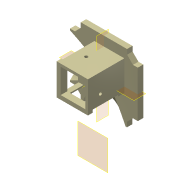
# Autodesk Inventor part: 20_Cube_Insert_Lightsheet_FEPTube_shifted_v3
Saved by Autodesk Inventor 2022 (Build 260153000, 153)
## iProperties
Created: 2019-07-01
Part Number: 20_Cube_Insert_Lightsheet_FEPTube_shifted_v3
Material: Generic
Document SubType Name: Modeling
Designer: diederichbenedict
Density: 1 g/cm^3
Appearance: Nylon 6
Author: diederichbenedict
Autodesk Inventor part; units mm, degrees
ref_plane "YZ Plane" through (0, 0, 0) normal (1, 0, 0) x (0, 1, 0)
ref_plane "XZ Plane" through (0, 0, 0) normal (0, 1, 0) x (-1, 0, 0)
ref_plane "Work Plane1" through (0, 0, 10) normal (0, 0, 1) x (1, 0, 0)
sketch "Sketch1" plane through (0, 0, 10) normal (0, 0, 1) x (1, 0, 0)
  line L0 (-4.029928, -0.353838) -> (-2.232156, 1.443934) construction
  arc A0 (-1.443934, 2.232156) -> (-2.232156, 1.443934) centre (-0.929928, 0.929928) ccw construction
  line L1 (-1.443934, 2.232156) -> (0.353838, 4.029928) construction
  line L2 (-37.829928, 42.829928) -> (-37.829928, 37.829928) construction
  line L3 (-37.829928, 37.829928) -> (-42.920801, 37.829928) construction
  line L4 (-37.829928, 42.213694) -> (-37.829928, 45.829928) construction
  line L5 (-37.829928, 45.829928) -> (-4.029928, 45.829928) construction
  line L6 (-4.029928, 45.829928) -> (-4.029928, 42.213694) construction
  line L7 (-4.029928, 4.029928) -> (0.353838, 4.029928)
  circle A1 centre (-20.929928, 20.929928) radius 17.5
  line L8 (-20.929928, 58.972273) -> (17.112417, 20.929928) construction
  line L9 (17.112417, 20.929928) -> (-20.929928, -17.112417) construction
  line L10 (-20.929928, -17.112417) -> (-58.972273, 20.929928) construction
  line L11 (-58.972273, 20.929928) -> (-20.929928, 58.972273) construction
  line L12 (-20.929928, 58.972273) -> (-20.929928, -17.112417) construction
  line L13 (17.112417, 20.929928) -> (-58.972273, 20.929928) construction
  line L14 (-20.929928, 58.972273) -> (32.870072, 58.972273) construction
  line L15 (-43.429928, 43.429928) -> (1.570072, 43.429928) construction
  line L16 (1.570072, 43.429928) -> (1.570072, -1.570072) construction
  line L17 (1.570072, -1.570072) -> (-43.429928, -1.570072) construction
  line L18 (-43.429928, -1.570072) -> (-43.429928, 43.429928) construction
  line L19 (-43.429928, 43.429928) -> (1.570072, -1.570072) construction
  line L20 (1.570072, 43.429928) -> (-43.429928, -1.570072) construction
  line L21 (-43.429928, 5.387583) -> (-43.429928, 36.472273)
  line L22 (-43.429928, 36.472273) -> (-36.472273, 43.429928)
  line L23 (-36.472273, 43.429928) -> (-5.387583, 43.429928)
  line L24 (-5.387583, 43.429928) -> (1.570072, 36.472273)
  line L25 (1.570072, 36.472273) -> (1.570072, 5.387583)
  line L26 (1.570072, 5.387583) -> (-5.387583, -1.570072)
  line L27 (-5.387583, -1.570072) -> (-36.472273, -1.570072)
  line L28 (-36.472273, -1.570072) -> (-43.429928, 5.387583)
  line L29 (-4.029928, 42.213694) -> (-37.829928, 42.213694)
  line L30 (-4.029928, -0.353838) -> (-4.029928, 4.029928)
  circle A2 centre (-20.929928, 20.929928) radius 1.5
  line L31 (-10.929928, 10.929928) -> (-30.929928, 10.929928) construction
  line L32 (-30.929928, 10.929928) -> (-30.929928, 30.929928) construction
  line L33 (-30.929928, 30.929928) -> (-10.929928, 30.929928) construction
  line L34 (-10.929928, 30.929928) -> (-10.929928, 10.929928) construction
  line L35 (-10.929928, 10.929928) -> (-30.929928, 30.929928) construction
  line L36 (-30.929928, 10.929928) -> (-10.929928, 30.929928) construction
  circle A3 centre (-30.929928, 30.929928) radius 1.4
  circle A4 centre (-30.929928, 10.929928) radius 1.4
  circle A5 centre (-10.929928, 10.929928) radius 1.4
  line L37 (-45.829928, 37.829928) -> (-42.072273, 37.829928) construction
  line L38 (-42.172273, 37.729928) -> (-45.829928, 37.729928)
  line L39 (-45.829928, 37.729928) -> (-45.829928, 4.129928)
  line L40 (-45.829928, 4.129928) -> (-42.172273, 4.129928)
  line L41 (-42.172273, 4.129928) -> (-42.172273, 37.729928)
  line L42 (-45.829928, 4.029928) -> (-42.072273, 4.029928) construction
  line L43 (-45.829928, 37.829928) -> (-42.072273, 37.829928)
  line L44 (-37.729928, 45.829928) -> (-4.129928, 45.829928)
  line L45 (-4.129928, 45.829928) -> (-4.129928, 42.172273)
  line L46 (-4.129928, 42.172273) -> (-37.729928, 42.172273)
  line L47 (-37.729928, 42.172273) -> (-37.729928, 45.829928)
  line L48 (0.470072, 37.829928) -> (0.470072, 4.029928) construction
  line L49 (0.470072, 4.029928) -> (3.970072, 4.029928) construction
  line L50 (3.970072, 37.829928) -> (3.970072, 4.029928) construction
  line L51 (0.470072, 37.829928) -> (3.970072, 37.829928) construction
  line L52 (-45.829928, -3.970072) -> (-4.029928, -3.970072) construction
  line L53 (0.312417, 37.729928) -> (3.970072, 37.729928)
  line L54 (3.970072, 37.729928) -> (3.970072, 4.129928)
  line L55 (3.970072, 4.129928) -> (0.312417, 4.129928)
  line L56 (0.312417, 4.129928) -> (0.312417, 37.729928)
  line L57 (-4.171349, -0.353838) -> (-37.729928, -0.353838)
  line L58 (-37.729928, -0.353838) -> (-37.729928, -3.970072)
  line L59 (-37.729928, -3.970072) -> (-4.171349, -3.970072)
  line L60 (-4.171349, -3.970072) -> (-4.171349, -0.353838)
  point P0 (-37.829928, 4.029928)
  dimension "d18" = 53.8
  dimension "d19" = 45
  dimension "d20" = 53.8
  dimension "d21" = 45
  dimension "d22" = 45
  dimension "d30" = 20
  dimension "d31" = 20
  dimension "d32" = 2.8
  dimension "d33" = 2.8
  dimension "d34" = 2.8
  dimension "d35" = 3
  dimension "d36" = 0.1
  dimension "d37" = 0.1
  dimension "d38" = 0.1
  dimension "d39" = 0.1
  constraints: 86 end point, 21 point on line, 14 parallel, 8 perpendicular, 7 horizontal, 7 midpoint, 4 centre point, 4 coincident, 1 equal length
  measures "d18" distance of L8.start L8.end
  measures "d19" angle of L8 L14
  measures "d20" distance of L8.end L9.end
  measures "d21" distance of L16.end L17.end
  measures "d22" distance of L15.end L16.end
  measures "d30" distance of L32.end L33.end
  measures "d31" distance of L31.end L32.end
  measures "d32" diameter of A3
  measures "d33" diameter of A4
  measures "d34" diameter of A5
  measures "d35" diameter of A2
  measures "d36" distance between parallel lines of L38 L43
  measures "d37" distance between parallel lines of L40 L42
  measures "d38" distance between parallel lines of L45 L6
  measures "d39" distance between parallel lines of L4 L47
sketch "Sketch1 outline for Extrusion1" plane through (0, 0, 10) normal (0, 0, 1) x (1, 0, 0)
  line L0 (-37.729928, -3.970072) -> (-4.171349, -3.970072)
  line L1 (-4.171349, -3.970072) -> (-4.171349, -0.353838)
  line L2 (0.312417, 4.129928) -> (-4.171349, -0.353838)
  line L3 (0.312417, 4.129928) -> (3.970072, 4.129928)
  line L4 (3.970072, 4.129928) -> (3.970072, 37.729928)
  line L5 (3.970072, 37.729928) -> (0.312417, 37.729928)
  line L6 (-4.129928, 42.172273) -> (0.312417, 37.729928)
  line L7 (-4.129928, 42.172273) -> (-4.129928, 45.829928)
  line L8 (-4.129928, 45.829928) -> (-37.729928, 45.829928)
  line L9 (-37.729928, 45.829928) -> (-37.729928, 42.172273)
  line L10 (-42.172273, 37.729928) -> (-37.729928, 42.172273)
  line L11 (-42.172273, 37.729928) -> (-45.829928, 37.729928)
  line L12 (-45.829928, 37.729928) -> (-45.829928, 4.129928)
  line L13 (-45.829928, 4.129928) -> (-42.172273, 4.129928)
  line L14 (-37.688507, -0.353838) -> (-42.172273, 4.129928)
  line L15 (-37.688507, -0.353838) -> (-37.729928, -0.353838)
  line L16 (-37.729928, -0.353838) -> (-37.729928, -3.970072)
extrude "Extrusion1" add sketch "Sketch1 outline for Extrusion1" along normal blind 3
sketch "Skizze4" plane through (0, 0, 13) normal (0, 0, 1) x (1, 0, 0)
  line L0 (-37.729928, 42.172273) -> (-42.172273, 37.729928)
  line L1 (-42.172273, 37.729928) -> (-45.829928, 37.729928)
  line L2 (-45.829928, 37.729928) -> (-45.829928, 4.129928) construction
  line L3 (-45.829928, 4.129928) -> (-42.172273, 4.129928)
  line L4 (-42.172273, 4.129928) -> (-37.688507, -0.353838)
  line L5 (-37.688507, -0.353838) -> (-37.729928, -0.353838)
  line L6 (-37.729928, -0.353838) -> (-37.729928, -3.970072)
  line L7 (-37.729928, -3.970072) -> (-4.171349, -3.970072) construction
  line L8 (-4.171349, -3.970072) -> (-4.171349, -0.353838)
  line L9 (-4.171349, -0.353838) -> (0.312417, 4.129928)
  line L10 (0.312417, 4.129928) -> (3.970072, 4.129928)
  line L11 (3.970072, 4.129928) -> (3.970072, 37.729928) construction
  line L12 (3.970072, 37.729928) -> (0.312417, 37.729928)
  line L13 (0.312417, 37.729928) -> (-4.129928, 42.172273)
  line L14 (-4.129928, 42.172273) -> (-4.129928, 45.829928)
  line L15 (-4.129928, 45.829928) -> (-37.729928, 45.829928) construction
  line L16 (-37.729928, 45.829928) -> (-37.729928, 42.172273)
  line L17 (-37.929928, 46.029928) -> (-3.929928, 46.029928) construction
  line L18 (-3.929928, 46.029928) -> (-3.929928, 42.255116)
  line L19 (-3.929928, 42.255116) -> (0.39526, 37.929928)
  line L20 (0.39526, 37.929928) -> (4.170072, 37.929928)
  line L21 (4.170072, 37.929928) -> (4.170072, 3.929928) construction
  line L22 (4.170072, 3.929928) -> (0.39526, 3.929928)
  line L23 (0.39526, 3.929928) -> (-3.971349, -0.436681)
  line L24 (-3.971349, -0.436681) -> (-3.971349, -4.170072)
  line L25 (-3.971349, -4.170072) -> (-37.929928, -4.170072) construction
  line L26 (-37.929928, -4.170072) -> (-37.929928, -0.39526)
  line L27 (-37.929928, -0.39526) -> (-42.255116, 3.929928)
  line L28 (-42.255116, 3.929928) -> (-46.029928, 3.929928)
  line L29 (-46.029928, 3.929928) -> (-46.029928, 37.929928) construction
  line L30 (-46.029928, 37.929928) -> (-42.255116, 37.929928)
  line L31 (-42.255116, 37.929928) -> (-37.929928, 42.255116)
  line L32 (-37.929928, 42.255116) -> (-37.929928, 46.029928)
  line L33 (-45.829928, 37.729928) -> (-45.829928, 37.929928)
  line L34 (-4.129928, 45.829928) -> (-37.729928, 45.829928)
  line L35 (-37.729928, 45.829928) -> (-37.929928, 45.829928)
  line L36 (-4.129928, 45.829928) -> (-3.929928, 45.829928)
  line L37 (3.970072, 37.729928) -> (3.970072, 37.929928)
  line L38 (3.970072, 4.129928) -> (3.970072, 37.729928)
  line L39 (3.970072, 4.129928) -> (3.970072, 3.929928)
  line L40 (-4.171349, -3.970072) -> (-3.971349, -3.970072)
  line L41 (-37.729928, -3.970072) -> (-37.929928, -3.970072)
  line L42 (-45.829928, 4.129928) -> (-45.829928, 3.929928)
  point P0 (0, 0)
  dimension "d40" = 0.2
  constraints: 48 end point, 12 point on line, 4 perpendicular, 15 other
  measures "d40" distance between parallel lines of L15 L17
sketch "Skizze4 outline for IM_offset" plane through (0, 0, 13) normal (0, 0, 1) x (1, 0, 0)
  line L0 (-3.929928, 45.829928) -> (-4.129928, 45.829928)
  line L1 (-3.929928, 42.255116) -> (-3.929928, 45.829928)
  line L2 (0.39526, 37.929928) -> (-3.929928, 42.255116)
  line L3 (3.970072, 37.929928) -> (0.39526, 37.929928)
  line L4 (3.970072, 37.729928) -> (3.970072, 37.929928)
  line L5 (0.312417, 37.729928) -> (3.970072, 37.729928)
  line L6 (-4.129928, 42.172273) -> (0.312417, 37.729928)
  line L7 (-4.129928, 45.829928) -> (-4.129928, 42.172273)
  line L8 (-42.172273, 37.729928) -> (-37.729928, 42.172273)
  line L9 (-45.829928, 37.729928) -> (-42.172273, 37.729928)
  line L10 (-45.829928, 37.929928) -> (-45.829928, 37.729928)
  line L11 (-42.255116, 37.929928) -> (-45.829928, 37.929928)
  line L12 (-37.929928, 42.255116) -> (-42.255116, 37.929928)
  line L13 (-37.929928, 45.829928) -> (-37.929928, 42.255116)
  line L14 (-37.729928, 45.829928) -> (-37.929928, 45.829928)
  line L15 (-37.729928, 42.172273) -> (-37.729928, 45.829928)
  line L16 (-45.829928, 4.129928) -> (-42.172273, 4.129928)
  line L17 (-42.172273, 4.129928) -> (-37.688507, -0.353838)
  line L18 (-37.688507, -0.353838) -> (-37.729928, -0.353838)
  line L19 (-37.729928, -0.353838) -> (-37.729928, -3.970072)
  line L20 (-37.729928, -3.970072) -> (-37.929928, -3.970072)
  line L21 (-37.929928, -3.970072) -> (-37.929928, -0.39526)
  line L22 (-37.929928, -0.39526) -> (-42.255116, 3.929928)
  line L23 (-42.255116, 3.929928) -> (-45.829928, 3.929928)
  line L24 (-45.829928, 3.929928) -> (-45.829928, 4.129928)
  line L25 (3.970072, 3.929928) -> (3.970072, 4.129928)
  line L26 (0.39526, 3.929928) -> (3.970072, 3.929928)
  line L27 (-3.971349, -0.436681) -> (0.39526, 3.929928)
  line L28 (-3.971349, -3.970072) -> (-3.971349, -0.436681)
  line L29 (-4.171349, -3.970072) -> (-3.971349, -3.970072)
  line L30 (-4.171349, -0.353838) -> (-4.171349, -3.970072)
  line L31 (0.312417, 4.129928) -> (-4.171349, -0.353838)
  line L32 (3.970072, 4.129928) -> (0.312417, 4.129928)
extrude "IM_offset" add sketch "Skizze4 outline for IM_offset" against normal up to surface (3 mm away)
ref_plane "Arbeitsebene5" through (-20.929928, 3.929928, 10) normal (1, 0, 0) x (0, 0, -1)
ref_plane "Arbeitsebene6" through (-37.929928, 20.929928, 10) normal (0, 1, 0) x (1, 0, 0)
sketch "Skizze25" plane through (0, 0, 13) normal (0, 0, 1) x (1, 0, 0)
  line L0 (3.970072, 3.929928) -> (3.970072, 37.929928)
  line L1 (3.970072, 37.929928) -> (0.39526, 37.929928)
  line L2 (0.39526, 37.929928) -> (-3.929928, 42.255116)
  line L3 (-3.929928, 42.255116) -> (-3.929928, 45.829928)
  line L4 (-3.929928, 45.829928) -> (-37.929928, 45.829928)
  line L5 (-37.929928, 45.829928) -> (-37.929928, 42.255116)
  line L6 (-37.929928, 42.255116) -> (-42.255116, 37.929928)
  line L7 (-42.255116, 37.929928) -> (-45.829928, 37.929928)
  line L8 (-45.829928, 37.929928) -> (-45.829928, 3.929928)
  line L9 (-42.255116, 3.929928) -> (-45.829928, 3.929928)
  line L10 (-37.929928, -0.39526) -> (-42.255116, 3.929928)
  line L11 (-37.929928, -3.970072) -> (-37.929928, -0.39526)
  line L12 (-3.971349, -3.970072) -> (-37.929928, -3.970072)
  line L13 (-3.971349, -3.970072) -> (-3.971349, -0.436681)
  line L14 (-3.971349, -0.436681) -> (0.39526, 3.929928)
  line L15 (0.39526, 3.929928) -> (3.970072, 3.929928)
  line L16 (-55.789928, 20.929928) -> (13.930072, 20.929928)
  line L17 (-25.929928, 36.929928) -> (-7.929928, 36.929928)
  line L18 (-7.929928, 36.929928) -> (-7.929928, 18.929928)
  line L19 (-7.929928, 18.929928) -> (-25.929928, 18.929928)
  line L20 (-25.929928, 18.929928) -> (-25.929928, 36.929928)
  line L21 (-25.929928, 36.929928) -> (-7.929928, 18.929928) construction
  line L22 (-7.929928, 36.929928) -> (-25.929928, 18.929928) construction
  line L23 (-20.929928, 55.789928) -> (-20.929928, -13.930072)
  line L24 (-5.929928, 38.929928) -> (-27.929928, 38.929928)
  line L25 (-27.929928, 38.929928) -> (-27.929928, 16.929928)
  line L26 (-27.929928, 16.929928) -> (-5.929928, 16.929928)
  line L27 (-5.929928, 16.929928) -> (-5.929928, 38.929928)
  line L28 (-27.929928, 16.929928) -> (-25.929928, 16.929928)
  line L29 (-25.929928, 16.929928) -> (-25.929928, 15.929928)
  line L30 (-25.929928, 15.929928) -> (-27.929928, 15.929928)
  line L31 (-27.929928, 15.929928) -> (-27.929928, 16.929928)
  point P0 (0, 0)
  point P1 (-16.929928, 27.929928)
  dimension "d194" = 18
  dimension "d195" = 18
  dimension "d196" = 2
  dimension "d197" = 5
  dimension "d198" = 2
  dimension "d210" = 2
  dimension "d211" = 1
  constraints: 28 end point, 6 parallel, 3 perpendicular, 2 horizontal, 2 midpoint, 3 other
  measures "d194" distance of L18.end L19.end
  measures "d195" distance of L17.end L18.end
  measures "d196" distance between parallel lines of L16 L19
  measures "d197" distance between parallel lines of L23 L20
  measures "d198" distance between parallel lines of L17 L24
  measures "d210" distance of L29.end L30.end
  measures "d211" distance of L28.end L29.end
sketch "Skizze25 outline for Extrusion21" plane through (0, 0, 13) normal (0, 0, 1) x (1, 0, 0)
  line L0 (-27.929928, 38.929928) -> (-27.929928, 16.929928)
  line L1 (-27.929928, 16.929928) -> (-27.929928, 15.929928)
  line L2 (-27.929928, 15.929928) -> (-25.929928, 15.929928)
  line L3 (-25.929928, 15.929928) -> (-25.929928, 16.929928)
  line L4 (-25.929928, 16.929928) -> (-5.929928, 16.929928)
  line L5 (-5.929928, 16.929928) -> (-5.929928, 38.929928)
  line L6 (-5.929928, 38.929928) -> (-27.929928, 38.929928)
  line L7 (-25.929928, 18.929928) -> (-25.929928, 36.929928)
  line L8 (-25.929928, 36.929928) -> (-7.929928, 36.929928)
  line L9 (-7.929928, 36.929928) -> (-7.929928, 18.929928)
  line L10 (-7.929928, 18.929928) -> (-25.929928, 18.929928)
extrude "Extrusion21" add sketch "Skizze25 outline for Extrusion21" along normal blind 25
ref_plane "Arbeitsebene9" through (0, 0, 42) normal (0, 0, 1) x (1, 0, 0)
sketch "Skizze28" plane through (-27.929928, 12.845867, 13) normal (-1, 0, 0) x (0, 0, 1)
  line L0 (51.2, 13.020711) -> (-25.1, 13.020711)
  line L1 (6, 6.084061) -> (22, 6.084061)
  line L2 (22, 6.084061) -> (22, 21.084061)
  line L3 (22, 21.084061) -> (6, 21.084061)
  line L4 (6, 21.084061) -> (6, 6.084061)
  line L5 (6, 6.084061) -> (22, 21.084061) construction
  line L6 (22, 6.084061) -> (6, 21.084061) construction
  line L7 (0, 24.084061) -> (25, 24.084061)
  line L8 (-3, -8.915939) -> (-3, 25.084061)
  line L9 (0, 6.084061) -> (25, 6.084061) construction
  point P0 (-13, -12.845867)
  point P1 (14, 13.584061)
  dimension "d206" = 16
  dimension "d207" = 15
  dimension "d209" = 17
  constraints: 14 end point, 2 horizontal, 2 midpoint, 2 parallel, 1 perpendicular, 1 point on line, 2 other
  measures "d206" distance of L3.end L2.end
  measures "d207" distance of L2.end L1.end
  measures "d209" distance from line of L8 point (14, 13.584)
sketch "Skizze28 outline for Extrusion24" plane through (-27.929928, 12.845867, 13) normal (-1, 0, 0) x (0, 0, 1)
  line L0 (6, 6.084061) -> (22, 6.084061)
  line L1 (6, 21.084061) -> (6, 6.084061)
  line L2 (22, 21.084061) -> (6, 21.084061)
  line L3 (22, 6.084061) -> (22, 21.084061)
extrude "Extrusion24" cut sketch "Skizze28 outline for Extrusion24" against normal blind 4
sketch "Skizze29" plane through (-32.315092, 16.929928, 13) normal (0, -1, 0) x (1, 0, 0)
  line L0 (26.385164, 0) -> (6.385164, 0)
  line L1 (26.385164, 0) -> (26.385164, 25)
  line L2 (6.385164, 25) -> (26.385164, 25)
  line L3 (6.385164, 0) -> (6.385164, 25)
  line L4 (4.385164, 22) -> (6.385164, 22)
  line L5 (4.385164, 6) -> (6.385164, 6)
  line L6 (8.385164, 22) -> (24.385164, 22)
  line L7 (24.385164, 22) -> (24.385164, 6)
  line L8 (24.385164, 6) -> (8.385164, 6)
  line L9 (8.385164, 6) -> (8.385164, 22)
  point P0 (32.315092, -13)
  point P1 (5.185164, 22)
  point P2 (5.185164, 6)
  dimension "d212" = 16
  dimension "d213" = 16
  dimension "d229" = 2
  constraints: 8 end point, 2 parallel, 1 horizontal, 1 perpendicular
  measures "d212" distance of L7.end L8.end
  measures "d213" distance of L6.end L7.end
  measures "d229" distance between parallel lines of L3 L9
sketch "Skizze29 outline for Extrusion25" plane through (-32.315092, 16.929928, 13) normal (0, -1, 0) x (1, 0, 0)
  line L0 (8.385164, 22) -> (8.385164, 6)
  line L1 (24.385164, 22) -> (8.385164, 22)
  line L2 (24.385164, 6) -> (24.385164, 22)
  line L3 (8.385164, 6) -> (24.385164, 6)
extrude "Extrusion25" cut sketch "Skizze29 outline for Extrusion25" against normal blind 4
ref_plane "Arbeitsebene7" through (-20.929928, 20.929928, 26.13) normal (-0.7071068, 0.7071068, 0) x (0.7071068, 0.7071068, 0)
sketch "Skizze32" plane through (0, 0, 10) normal (0, 0, -1) x (-1, 0, 0)
  line L0 (3.971349, -3.970072) -> (37.929928, -3.970072)
  line L1 (37.929928, -3.970072) -> (37.929928, -0.39526)
  line L2 (37.929928, -0.39526) -> (42.255116, 3.929928)
  line L3 (42.255116, 3.929928) -> (45.829928, 3.929928)
  line L4 (45.829928, 3.929928) -> (45.829928, 37.929928)
  line L5 (45.829928, 37.929928) -> (42.255116, 37.929928)
  line L6 (42.255116, 37.929928) -> (37.929928, 42.255116)
  line L7 (37.929928, 42.255116) -> (37.929928, 45.829928)
  line L8 (37.929928, 45.829928) -> (3.929928, 45.829928)
  line L9 (3.929928, 45.829928) -> (3.929928, 42.255116)
  line L10 (3.929928, 42.255116) -> (-0.39526, 37.929928)
  line L11 (-0.39526, 37.929928) -> (-3.970072, 37.929928)
  line L12 (-3.970072, 37.929928) -> (-3.970072, 3.929928)
  line L13 (-3.970072, 3.929928) -> (-0.39526, 3.929928)
  line L14 (-0.39526, 3.929928) -> (3.971349, -0.436681)
  line L15 (3.971349, -0.436681) -> (3.971349, -3.970072)
  point P0 (0, 0)
sketch "Skizze32 outline for Extrusion28" plane through (0, 0, 10) normal (0, 0, -1) x (-1, 0, 0)
  line L0 (3.971349, -3.970072) -> (37.929928, -3.970072)
  line L1 (3.971349, -0.436681) -> (3.971349, -3.970072)
  line L2 (-0.39526, 3.929928) -> (3.971349, -0.436681)
  line L3 (-3.970072, 3.929928) -> (-0.39526, 3.929928)
  line L4 (-3.970072, 37.929928) -> (-3.970072, 3.929928)
  line L5 (-0.39526, 37.929928) -> (-3.970072, 37.929928)
  line L6 (3.929928, 42.255116) -> (-0.39526, 37.929928)
  line L7 (3.929928, 45.829928) -> (3.929928, 42.255116)
  line L8 (37.929928, 45.829928) -> (3.929928, 45.829928)
  line L9 (37.929928, 42.255116) -> (37.929928, 45.829928)
  line L10 (42.255116, 37.929928) -> (37.929928, 42.255116)
  line L11 (45.829928, 37.929928) -> (42.255116, 37.929928)
  line L12 (45.829928, 3.929928) -> (45.829928, 37.929928)
  line L13 (42.255116, 3.929928) -> (45.829928, 3.929928)
  line L14 (37.929928, -0.39526) -> (42.255116, 3.929928)
  line L15 (37.929928, -3.970072) -> (37.929928, -0.39526)
extrude "Extrusion28" add sketch "Skizze32 outline for Extrusion28" along normal blind 1
sketch "Skizze33" plane through (-37.929928, -3.970072, 13) normal (0, -1, 0) x (1, 0, 0)
  line L0 (0.03, -3.97) -> (0.03, 30.13) construction
  line L1 (33.958579, 0) -> (33.958579, -4)
  line L2 (33.958579, 0) -> (0, 0)
  line L3 (0, 0) -> (0, -4)
  line L4 (33.958579, -4) -> (0, -4)
  circle A0 centre (16.994289, 12.964289) radius 16.964289
  circle A1 centre (16.994289, 12.964289) radius 20.476427
  point P0 (37.929928, -13)
  point P1 (18.664772, 13.05)
  constraints: 3 tangent, 2 centre point
sketch "Skizze33 outline for Extrusion29" plane through (-37.929928, -3.970072, 13) normal (0, -1, 0) x (1, 0, 0)
  circle A0 centre (16.994289, 12.964289) radius 20.476427
extrude "Extrusion29" cut sketch "Skizze33 outline for Extrusion29" against normal blind 17 draft -20
sketch "Skizze36" plane through (-25.929928, 36.929928, 13) normal (0, -1, 0) x (1, 0, 0)
  line L0 (18, 0) -> (0, 0) projected
  line L1 (18, 0) -> (18, 25) projected
  line L2 (0, 25) -> (18, 25) projected
  line L3 (0, 0) -> (0, 25) projected
  line L4 (18, 0) -> (2, 0)
  line L5 (2, 0) -> (2, 16)
  line L6 (2, 16) -> (18, 16)
  line L7 (18, 16) -> (18, 0)
  point P0 (25.929928, -13)
  dimension "d214" = 16
  dimension "d215" = 16
  constraints: 8 end point, 2 parallel, 1 horizontal, 1 perpendicular
  measures "d214" distance of L5.end L6.end
  measures "d215" distance of L4.end L5.end
sketch "Skizze36 outline for Extrusion32" plane through (-25.929928, 36.929928, 13) normal (0, -1, 0) x (1, 0, 0)
  line L0 (18, 16) -> (2, 16)
  line L1 (18, 0) -> (18, 16)
  line L2 (2, 0) -> (18, 0)
  line L3 (2, 16) -> (2, 0)
extrude "Extrusion32" add sketch "Skizze36 outline for Extrusion32" along normal blind 14
sketch "Skizze37" plane through (-27.929928, 38.929928, 13) normal (0, 1, 0) x (1, 0, 0)
  line L0 (0, 0) -> (22, 0) projected
  line L1 (0, 0) -> (0, -25) projected
  line L2 (22, -25) -> (0, -25) projected
  line L3 (22, 0) -> (22, -25) projected
  line L4 (7, 20.6) -> (7, -32.6) projected
  circle A0 centre (7, -13) radius 1.15
  line L5 (-10, 4) -> (24, 4) projected
  point P0 (27.929928, 13)
  dimension "d218" = 2.3
  dimension "d219" = 17
  constraints: 1 centre point, 1 point on line
  measures "d218" diameter of A0
  measures "d219" distance from line of A0.centre L5
sketch "Skizze37 outline for Extrusion33" plane through (-27.929928, 38.929928, 13) normal (0, 1, 0) x (1, 0, 0)
  circle A0 centre (7, -13) radius 1.15
extrude "Extrusion33" cut sketch "Skizze37 outline for Extrusion33" against normal through all
sketch "Skizze38" plane through (-5.929928, 16.929928, 13) normal (1, 0, 0) x (0, 0, -1)
  line L0 (-14.15, 22) -> (-14.15, 6)
  line L1 (-11.85, 22) -> (-11.85, 6)
  circle A0 centre (-17.462329, 8.158818) radius 1.15
  point P0 (13, -16.929928)
  dimension "d222" = 2.3
  constraints: 1 centre point
  measures "d222" diameter of A0
sketch "Skizze38 outline for Extrusion34" plane through (-5.929928, 16.929928, 13) normal (1, 0, 0) x (0, 0, -1)
  circle A0 centre (-17.462329, 8.158818) radius 1.15
extrude "Extrusion34" cut sketch "Skizze38 outline for Extrusion34" against normal through all
mirror "Spiegeln4" about plane through (-20.929928, 20.929928, 26.13) normal (-0.7071068, 0.7071068, 0) of "Extrusion29"
sketch "Skizze39" plane through (-27.929928, 15.929928, 13) normal (-1, 0, 0) x (0, 0, 1)
  line L0 (6, 18) -> (22, 18) projected
  line L1 (22, 18) -> (22, 3) projected
  line L2 (22, 3) -> (6, 3) projected
  line L3 (6, 3) -> (6, 18) projected
  line L4 (0, 0) -> (0, 23) projected
  line L5 (0, 0) -> (25, 0) projected
  line L6 (25, 23) -> (25, 0) projected
  line L7 (0, 23) -> (25, 23) projected
  line L8 (23.25, 19.75) -> (4.75, 19.75)
  line L9 (4.75, 19.75) -> (4.75, 1.25)
  line L10 (4.75, 1.25) -> (23.25, 1.25)
  line L11 (23.25, 1.25) -> (23.25, 19.75)
  line L12 (23.25, 19.75) -> (4.75, 1.25) construction
  line L13 (4.75, 19.75) -> (23.25, 1.25) construction
  point P0 (-13, -15.929928)
  point P1 (14, 10.5)
  dimension "d225" = 18.5
  dimension "d226" = 18.5
  constraints: 12 end point, 2 midpoint, 2 parallel, 1 horizontal, 1 perpendicular
  measures "d225" distance of L10.end L9.end
  measures "d226" distance of L9.end L8.end
sketch "Skizze39 outline for Extrusion35" plane through (-27.929928, 15.929928, 13) normal (-1, 0, 0) x (0, 0, 1)
  line L0 (23.25, 19.75) -> (4.75, 19.75)
  line L1 (23.25, 1.25) -> (23.25, 19.75)
  line L2 (4.75, 1.25) -> (23.25, 1.25)
  line L3 (4.75, 19.75) -> (4.75, 1.25)
extrude "Extrusion35" cut sketch "Skizze39 outline for Extrusion35" against normal blind 0.5
sketch "Skizze40" plane through (-25.929928, 16.929928, 13) normal (0, -1, 0) x (1, 0, 0)
  line L0 (18, 22) -> (18, 6) projected
  line L1 (18, 6) -> (2, 6) projected
  line L2 (2, 6) -> (2, 22) projected
  line L3 (2, 22) -> (18, 22) projected
  line L4 (20, 0) -> (0, 0) projected
  line L5 (20, 0) -> (20, 25) projected
  line L6 (0, 25) -> (20, 25) projected
  line L7 (0, 0) -> (0, 25) projected
  line L8 (19.25, 23.25) -> (19.25, 4.75)
  line L9 (19.25, 4.75) -> (0.75, 4.75)
  line L10 (0.75, 4.75) -> (0.75, 23.25)
  line L11 (0.75, 23.25) -> (19.25, 23.25)
  line L12 (0, 0) -> (0, 25) projected
  line L13 (0, 23.25) -> (0.75, 23.25)
  line L14 (0.75, 23.25) -> (0.75, 4.75)
  line L15 (0.75, 4.75) -> (0, 4.75)
  line L16 (0, 4.75) -> (0, 23.25)
  line L17 (20, 0) -> (20, 25) projected
  line L18 (19.25, 23.25) -> (20, 23.25)
  line L19 (20, 23.25) -> (20, 4.75)
  line L20 (20, 4.75) -> (19.25, 4.75)
  line L21 (19.25, 4.75) -> (19.25, 23.25)
  point P0 (25.929928, -13)
  point P1 (0, 4.75)
  point P2 (20, 4.75)
  point P3 (0.75, 23.25)
  dimension "d230" = 18.5
  constraints: 24 end point, 4 parallel, 3 point on line, 2 horizontal, 2 perpendicular, 3 other
  measures "d230" distance between parallel lines of L8 L10
sketch "Skizze40 outline for Extrusion36" plane through (-25.929928, 16.929928, 13) normal (0, -1, 0) x (1, 0, 0)
  line L0 (0, 4.75) -> (0.75, 4.75)
  line L1 (0, 23.25) -> (0, 4.75)
  line L2 (0.75, 4.75) -> (19.25, 4.75)
  line L3 (0.75, 23.25) -> (0, 23.25)
  line L4 (19.25, 4.75) -> (20, 4.75)
  line L5 (19.25, 23.25) -> (0.75, 23.25)
  line L6 (20, 4.75) -> (20, 23.25)
  line L7 (20, 23.25) -> (19.25, 23.25)
  line L8 (18, 22) -> (18, 6)
  line L9 (2, 22) -> (18, 22)
  line L10 (2, 6) -> (2, 22)
  line L11 (18, 6) -> (2, 6)
extrude "Extrusion36" cut sketch "Skizze40 outline for Extrusion36" against normal blind 1
sketch "Skizze41" plane through (0, 0, 38) normal (0, 0, 1) x (1, 0, 0)
  line L0 (-25.929928, 16.929928) -> (-5.929928, 16.929928)
  line L1 (-5.929928, 16.929928) -> (-5.929928, 38.929928)
  line L2 (-5.929928, 38.929928) -> (-27.929928, 38.929928)
  line L3 (-27.929928, 38.929928) -> (-27.929928, 15.929928)
  line L4 (-27.929928, 15.929928) -> (-25.929928, 15.929928)
  line L5 (-25.929928, 15.929928) -> (-25.929928, 16.929928)
  line L6 (-25.929928, 18.929928) -> (-25.929928, 36.929928)
  line L7 (-25.929928, 36.929928) -> (-7.929928, 36.929928)
  line L8 (-7.929928, 36.929928) -> (-7.929928, 18.929928)
  line L9 (-7.929928, 18.929928) -> (-25.929928, 18.929928)
  line L10 (-25.929928, 38.929928) -> (-28.929928, 38.929928)
  line L11 (-28.929928, 38.929928) -> (-28.929928, 15.929928)
  line L12 (-28.929928, 15.929928) -> (-25.929928, 15.929928)
  line L13 (-25.929928, 15.929928) -> (-25.929928, 38.929928)
  line L14 (-25.929928, 15.929928) -> (-5.929928, 15.929928)
  line L15 (-5.929928, 15.929928) -> (-5.929928, 18.929928)
  line L16 (-5.929928, 18.929928) -> (-25.929928, 18.929928)
  line L17 (-25.929928, 18.929928) -> (-25.929928, 15.929928)
  point P0 (0, 0)
  dimension "d233" = 3
  constraints: 16 end point, 4 parallel, 2 horizontal, 2 perpendicular, 2 point on line
  measures "d233" distance of L12.end L11.end
sketch "Skizze41 outline for Extrusion37" plane through (0, 0, 38) normal (0, 0, 1) x (1, 0, 0)
  line L0 (-5.929928, 38.929928) -> (-27.929928, 38.929928)
  line L1 (-5.929928, 16.929928) -> (-5.929928, 38.929928)
  line L2 (-27.929928, 38.929928) -> (-28.929928, 38.929928)
  line L3 (-5.929928, 15.929928) -> (-5.929928, 16.929928)
  line L4 (-28.929928, 38.929928) -> (-28.929928, 15.929928)
  line L5 (-25.929928, 15.929928) -> (-5.929928, 15.929928)
  line L6 (-28.929928, 15.929928) -> (-27.929928, 15.929928)
  line L7 (-27.929928, 15.929928) -> (-25.929928, 15.929928)
  line L8 (-25.929928, 36.929928) -> (-7.929928, 36.929928)
  line L9 (-25.929928, 18.929928) -> (-25.929928, 36.929928)
  line L10 (-7.929928, 18.929928) -> (-25.929928, 18.929928)
  line L11 (-7.929928, 36.929928) -> (-7.929928, 18.929928)
extrude "Extrusion37" add sketch "Skizze41 outline for Extrusion37" along normal mid plane 3.5
chamfer "Fase3" distance 2 angle 45 1 edges at (-15.9299, 15.9299, 36.25)
body "Solid1"
